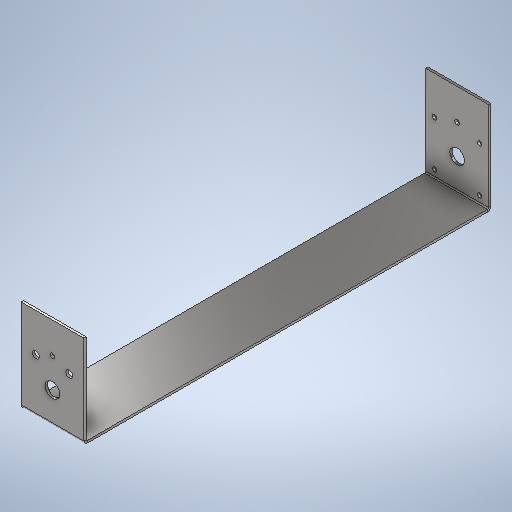
# Autodesk Inventor part: Bracket (Sheet Metal)
Saved by Autodesk Inventor 2025.1 (Build 291241020, 241B)
## iProperties
Created: 2025-04-17
Part Number: Bracket (Sheet Metal)
Material: Steel, Carbon
Document SubType Name: Sheet Metal
Designer: aidan
Density: 7.85 g/cm^3
Sheet Metal Rule: Default
Appearance: Semi-Polished
Author: aidan
Autodesk Inventor part; units mm, degrees
ref_plane "YZ Plane" through (0, 0, 0) normal (1, 0, 0) x (0, 1, 0)
ref_plane "XZ Plane" through (0, 0, 0) normal (0, 1, 0) x (-1, 0, 0)
ref_plane "XY Plane" through (0, 0, 0) normal (0, 0, 1) x (1, 0, 0)
sketch "Sketch2" plane through (0, 0, 0) normal (0, 1, 0) x (-1, 0, 0)
  line L0 (-21.59, -138.1125) -> (21.59, -138.1125)
  line L1 (21.59, -138.1125) -> (21.59, 138.1125)
  line L2 (21.59, 138.1125) -> (-21.59, 138.1125)
  line L3 (-21.59, 138.1125) -> (-21.59, -138.1125)
  line L4 (-21.59, -138.1125) -> (21.59, 138.1125) construction
  line L5 (21.59, -138.1125) -> (-21.59, 138.1125) construction
  point P0 (0, 0)
  dimension "d2" = 43.18
  dimension "d3" = 276.225
  measures "d2" distance of L1.end L2.end
  measures "d3" distance of L0.end L1.end
extrude "Plate1" add sketch "Sketch2" along normal blind 1.5875
sketch "Sketch3" plane through (21.59, 0, 139.7) normal (0, 0, -1) x (-1, 0, 0)
  line L0 (43.18, 0) -> (0, 0)
  line L1 (0, 0) -> (0, 63.5)
  line L2 (0, 63.5) -> (43.18, 63.5)
  line L3 (43.18, 63.5) -> (43.18, 0)
  constraints: 8 end point
edge flange "Flange1" height 63.5 angle 90 thickness 1.5875 bend radius 0.762 thickness toward (0, 0, -1) relief straight relief width 1.5875 relief depth 0.7937 edges at (0, 1.5875, 138.1125) wall of the first edge with corners at (-21.59, 0, 139.7) (21.59, 0, 139.7) (21.59, 63.5, 139.7) (-21.59, 63.5, 139.7)
bend "Bend1"
corner "Corner1"
sketch "Sketch4" plane through (-21.59, 0, -139.7) normal (0, 0, 1) x (1, 0, 0)
  line L0 (43.18, 0) -> (0, 0)
  line L1 (0, 0) -> (0, 63.5)
  line L2 (0, 63.5) -> (43.18, 63.5)
  line L3 (43.18, 63.5) -> (43.18, 0)
  constraints: 8 end point
edge flange "Flange2" height 63.5 angle 90 thickness 1.5875 bend radius 0.762 thickness toward (0, 0, 1) relief straight relief width 1.5875 relief depth 0.7937 edges at (0, 1.5875, -138.1125) wall of the first edge with corners at (21.59, 0, -139.7) (-21.59, 0, -139.7) (-21.59, 63.5, -139.7) (21.59, 63.5, -139.7)
bend "Bend2"
corner "Corner2"
sketch "Sketch5" plane through (-21.59, 63.5, 139.7) normal (0, 0, 1) x (1, 0, 0)
  line L0 (43.18, 0) -> (43.18, -61.1505) projected
  line L1 (43.18, -61.1505) -> (0, -61.1505) projected
  line L2 (0, -61.1505) -> (43.18, -61.1505) projected
  line L3 (0, -61.9125) -> (43.18, -61.9125) projected
  point P0 (21.59, -63.5)
  point P1 (21.59, -21.2725)
  point P2 (21.59, -41.5925)
  point P3 (21.59, -61.1505)
  dimension "d37" = 20.32
  dimension "d38" = 21.59
  dimension "d39" = 21.59
  dimension "d83" = 20.32
  constraints: 1 midpoint
  measures "d37" distance of point (21.59, -21.273) point (21.59, -41.593)
  measures "d38" distance from line of L0 point (21.59, -41.593)
  measures "d39" distance from line of L0 point (21.59, -21.273)
  measures "d83" distance from line of L3 point (21.59, -41.593)
hole "Hole2" at (0, 21.9075, 139.7) at (0, 42.2275, 139.7) direction (0, 0, -1) diameter 3.175 depth 279.4 tip angle 118
sketch "Sketch7" plane through (-21.59, 63.5, 139.7) normal (0, 0, 1) x (1, 0, 0)
  circle A0 centre (21.59, -41.5925) radius 1.5875 projected
  point P0 (21.59, -63.5)
  constraints: 1 coincident
hole "Hole3" at (0, 21.9075, 139.7) direction (0, 0, -1) diameter 10.1092 depth 279.4 tip angle 118
sketch "Sketch8" plane through (-21.59, 63.5, 139.7) normal (0, 0, 1) x (1, 0, 0)
  line L0 (0, -61.1505) -> (0, 0) projected
  line L1 (43.18, 0) -> (43.18, -61.1505) projected
  circle A0 centre (21.59, -41.5925) radius 5.0546 projected
  point P0 (21.59, -63.5)
  point P1 (10.16, -26.3525)
  point P2 (33.02, -26.3525)
  dimension "d54" = 10.16
  dimension "d55" = 10.16
  dimension "d56" = 15.24
  dimension "d57" = 15.24
  measures "d54" distance from line of L0 point (10.16, -26.353)
  measures "d55" distance from line of L1 point (33.02, -26.353)
  measures "d56" vertical distance of point (10.16, -26.353) A0.centre
  measures "d57" vertical distance of point (33.02, -26.353) A0.centre
hole "Hole4" at (-11.43, 37.1475, 139.7) at (11.43, 37.1475, 139.7) direction (0, 0, -1) diameter 4.7625 depth 1.5875 tip angle 118
sketch "Sketch9" plane through (21.59, 63.5, -139.7) normal (0, 0, -1) x (-1, 0, 0)
  circle A0 centre (21.59, -41.5925) radius 5.0546 projected
  point P0 (21.59, -63.5)
  point P1 (37.084, -26.0985)
  point P2 (37.084, -57.0865)
  point P3 (6.096, -57.0865)
  point P4 (6.096, -26.0985)
  dimension "d65" = 15.494
  dimension "d68" = 15.494
  dimension "d69" = 15.494
  dimension "d70" = 15.494
  dimension "d71" = 15.494
  dimension "d72" = 15.494
  dimension "d73" = 15.494
  dimension "d74" = 15.494
  measures "d65" horizontal distance of point (6.096, -57.087) A0.centre
  measures "d68" horizontal distance of point (6.096, -57.087) A0.centre
  measures "d69" horizontal distance of point (6.096, -26.099) A0.centre
  measures "d70" horizontal distance of A0.centre point (6.096, -26.099)
  measures "d71" horizontal distance of A0.centre point (37.084, -26.099)
  measures "d72" horizontal distance of A0.centre point (37.084, -26.099)
  measures "d73" horizontal distance of point (37.084, -57.087) A0.centre
  measures "d74" horizontal distance of A0.centre point (37.084, -57.087)
hole "Hole5" at (-15.494, 37.4015, -139.7) at (-15.494, 6.4135, -139.7) at (15.494, 6.4135, -139.7) at (15.494, 37.4015, -139.7) direction (0, 0, 1) diameter 3.175 depth 1.5875 tip angle 118
equation "\"d4\" = Thickness"
equation "\"d5\" = BendReliefWidth"
equation "\"d6\" = BendReliefDepth"
equation "\"d7\" = MinimumRemnant"
equation "\"d8\" = TransitionRadius"
equation "\"d12\" = CornerReliefSize"
equation "\"d13\" = GapSize"
equation "\"d14\" = JacobiRadiusSize"
equation "\"d15\" = BendReliefWidth"
equation "\"d16\" = BendReliefDepth"
equation "\"d17\" = MinimumRemnant"
equation "\"d18\" = TransitionRadius"
equation "\"d22\" = CornerReliefSize"
equation "\"d23\" = GapSize"
equation "\"d24\" = JacobiRadiusSize"
equation "\"BendRadius\" = Thickness"
equation "\"BendReliefWidth\" = Thickness"
equation "\"BendReliefDepth\" = 0.5 * Thickness"
equation "\"CornerReliefSize\" = 4 * Thickness"
equation "\"MinimumRemnant\" = 2 * Thickness"
equation "\"TransitionRadius\" = BendRadius"
equation "\"JacobiRadiusSize\" = BendRadius"
equation "\"GapSize\" = Thickness"
equation "\"Thickness\" = 1.5875"
body "Solid1"
